Autodesk Fusion 360 part; units mm, degrees
(part 3 of 3)
  point P128 (211, 51)
  point P129 (218.0002, 50.9466)
  point P130 (228.5461, 44.9647)
  point P131 (221.5464, 44.9113)
  point P132 (225, 51)
  point P133 (225, 51)
  point P134 (225, 51)
  point P135 (134.0002, 62.9466)
  point P136 (144.5461, 56.9647)
  point P137 (137.5464, 56.9113)
  point P138 (141, 63)
  point P139 (141, 63)
  point P140 (141, 63)
  point P141 (148.0002, 62.9466)
  point P142 (158.5461, 56.9647)
  point P143 (151.5464, 56.9113)
  point P144 (155, 63)
  point P145 (155, 63)
  point P146 (155, 63)
  point P147 (162.0002, 62.9466)
  point P148 (172.5461, 56.9647)
  point P149 (165.5464, 56.9113)
  point P150 (169, 63)
  point P151 (169, 63)
  point P152 (169, 63)
  point P153 (190.0002, 62.9466)
  point P154 (200.5461, 56.9647)
  point P155 (193.5464, 56.9113)
  point P156 (197, 63)
  point P157 (197, 63)
  point P158 (197, 63)
  point P159 (204.0002, 62.9466)
  point P160 (214.5461, 56.9647)
  point P161 (207.5464, 56.9113)
  point P162 (211, 63)
  point P163 (211, 63)
  point P164 (211, 63)
  point P165 (218.0002, 62.9466)
  point P166 (228.5461, 56.9647)
  point P167 (221.5464, 56.9113)
  point P168 (225, 63)
  point P169 (225, 63)
  point P170 (225, 63)
  point P171 (134.0002, 74.9466)
  point P172 (144.5461, 68.9647)
  point P173 (137.5464, 68.9113)
  point P174 (141, 75)
  point P175 (141, 75)
  point P176 (141, 75)
  point P177 (148.0002, 74.9466)
  point P178 (158.5461, 68.9647)
  point P179 (151.5464, 68.9113)
  point P180 (155, 75)
  point P181 (155, 75)
  point P182 (155, 75)
  point P183 (162.0002, 74.9466)
  point P184 (172.5461, 68.9647)
  point P185 (165.5464, 68.9113)
  point P186 (169, 75)
  point P187 (169, 75)
  point P188 (169, 75)
  point P189 (176.0002, 74.9466)
  point P190 (186.5461, 68.9647)
  point P191 (179.5464, 68.9113)
  point P192 (183, 75)
  point P193 (183, 75)
  point P194 (183, 75)
  point P195 (190.0002, 74.9466)
  point P196 (200.5461, 68.9647)
  point P197 (193.5464, 68.9113)
  point P198 (197, 75)
  point P199 (197, 75)
  point P200 (197, 75)
  point P201 (204.0002, 74.9466)
  point P202 (214.5461, 68.9647)
  point P203 (207.5464, 68.9113)
  point P204 (211, 75)
  point P205 (211, 75)
  point P206 (211, 75)
  point P207 (218.0002, 74.9466)
  point P208 (228.5461, 68.9647)
  point P209 (221.5464, 68.9113)
  point P210 (225, 75)
  point P211 (225, 75)
  point P212 (225, 75)
  point P213 (134.0002, 86.9466)
  point P214 (144.5461, 80.9647)
  point P215 (137.5464, 80.9113)
  point P216 (141, 87)
  point P217 (141, 87)
  point P218 (141, 87)
  point P219 (148.0002, 86.9466)
  point P220 (158.5461, 80.9647)
  point P221 (151.5464, 80.9113)
  point P222 (155, 87)
  point P223 (155, 87)
  point P224 (155, 87)
  point P225 (162.0002, 86.9466)
  point P226 (172.5461, 80.9647)
  point P227 (165.5464, 80.9113)
  point P228 (169, 87)
  point P229 (169, 87)
  point P230 (169, 87)
  point P231 (176.0002, 86.9466)
  point P232 (186.5461, 80.9647)
  point P233 (179.5464, 80.9113)
  point P234 (183, 87)
  point P235 (183, 87)
  point P236 (183, 87)
  point P237 (190.0002, 86.9466)
  point P238 (200.5461, 80.9647)
  point P239 (193.5464, 80.9113)
  point P240 (197, 87)
  point P241 (197, 87)
  point P242 (197, 87)
  point P243 (204.0002, 86.9466)
  point P244 (214.5461, 80.9647)
  point P245 (207.5464, 80.9113)
  point P246 (211, 87)
  point P247 (211, 87)
  point P248 (211, 87)
  point P249 (218.0002, 86.9466)
  point P250 (228.5461, 80.9647)
  point P251 (221.5464, 80.9113)
  point P252 (225, 87)
  point P253 (225, 87)
  point P254 (225, 87)
  point P255 (134.0002, 98.9466)
  point P256 (144.5461, 92.9647)
  point P257 (137.5464, 92.9113)
  point P258 (141, 99)
  point P259 (141, 99)
  point P260 (141, 99)
  point P261 (148.0002, 98.9466)
  point P262 (158.5461, 92.9647)
  point P263 (151.5464, 92.9113)
  point P264 (155, 99)
  point P265 (155, 99)
  point P266 (155, 99)
  point P267 (162.0002, 98.9466)
  point P268 (172.5461, 92.9647)
  point P269 (165.5464, 92.9113)
  point P270 (169, 99)
  point P271 (169, 99)
  point P272 (169, 99)
  point P273 (176.0002, 98.9466)
  point P274 (186.5461, 92.9647)
  point P275 (179.5464, 92.9113)
  point P276 (183, 99)
  point P277 (183, 99)
  point P278 (183, 99)
  point P279 (190.0002, 98.9466)
  point P280 (200.5461, 92.9647)
  point P281 (193.5464, 92.9113)
  point P282 (197, 99)
  point P283 (197, 99)
  point P284 (197, 99)
  point P285 (204.0002, 98.9466)
  point P286 (214.5461, 92.9647)
  point P287 (207.5464, 92.9113)
  point P288 (211, 99)
  point P289 (211, 99)
  point P290 (211, 99)
  point P291 (218.0002, 98.9466)
  point P292 (228.5461, 92.9647)
  point P293 (221.5464, 92.9113)
  point P294 (225, 99)
  point P295 (225, 99)
  point P296 (225, 99)
  dimension "d52" = 75
  dimension "d55" = 3
  dimension "d56" = 3
  dimension "d57" = 3
  dimension "d58" = 3
  dimension "d59" = 1
  dimension "d60" = 1
  dimension "d61" = 1
  dimension "d62" = 1
  dimension "d63" = 1
  dimension "d64" = 60
  dimension "d65" = 60
  dimension "d68" = 42
  dimension "d69" = 36
  constraint coincident L10.end L11.start
  constraint coincident L13.end L15.start
  constraint coincident P5 A0.centre
  constraint parallel L54 L71
  constraint parallel L63 L65
  constraint coincident A0 L77.end
  constraint perpendicular L58 L77
  measures "d52" diameter of A0
  measures "d55" distance of P5 L58
  measures "d56" distance of P6 L64
  measures "d57" distance of P7 L70
  measures "d58" distance of P8 L76
  measures "d59" distance of L58 L64
  measures "d60" distance of L54 L71
  measures "d61" distance of L63 L65
  measures "d62" distance of L53 L70
  measures "d63" distance of L69 L72
  measures "d64" distance of P5 L52
  measures "d65" distance of L23 P5
extrude "Extrude5" add sketch "Sketch4" along normal blind 6 separate body contours A0 L127 L130 L147 L151 L154 L155 L159 L162 L168 L169 L171 L175 L178 L179 L183 L186 L192 L193 L271 L274 L278 L287 L291 L292 L293 L294 L296 L304 L305 L309 L349 L350 L356 L364 L365 L367 L368 L370 L377 L378 L381 L382 L438 L447 L448 L449 L451 L453 L456 L457 L541 L542 L548 L557 L561 L563 L567 L577 L588 L604 L605 L609 L615 L619 L624 L625 L704 L705 L707 L711 L715 L717 L721 L722 L732 L748 L749 L753 L759 L763 L768 L872 L873 L875 L883 L885 L889 L890 L913 L914 L922 L923 L928 L929 L932 L933 L1012 L1014 L1015 L1016 L1020 L1022 L1024 L1025 L1073 L1080 L1088 L1090 L1092 L1100 L1101 L1106 L1107 L1110 L1111 L1117 L1119 L1126 L1127 L1130 L1131 L1132 L1135 L1141 L1143 L1144 L1145 L1146 L1150 L1151 L1152 L1154 L1155 L1156 L1160 L1164 L1172 L1182 makes body 5
extrude "Extrude6" add sketch "Sketch4" along normal blind 6 contours L0 L1 L2 L3 L4 L5 L6 L7 L8 L9 L10 L11 L12 L13 L14 L15 L16 L17 L18 L19 L20 L21 L22 L23 L24 L25 L26 L27 L28 L29 L30 L31 L32 L33 L34 L35 L36 L37 L38 L39 L40 L41 L42 L43 L44 L45 L46 L47 L48 L49 L50 L51 | A0 L1091 L1094 L1102 L1106 L1111 | A0 L276 L277 L278 L284 L292 | A0 L1074 L1075 L1080 L1088 L1089 | A0 L274 L282 L286 L287 | A0 L914 L917 L924 L928 | A0 L440 L448 L453 L458 | A0 L915 L923 L927 L932 | A0 L441 L443 L451 L457 | A0 L753 L755 L759 L769 | A0 L588 L589 L590 L596 L605 | A0 L732 L733 L734 L740 L749 | A0 L609 L611 L625 | L79 L82 L90 L94 L95 L99 | L81 L83 L87 L91 L96 L97 | L246 L248 L256 L257 L261 L266 | L247 L250 L258 L262 L263 L267 | L249 L251 L255 L259 L264 L265 | L252 L253 L254 L260 L268 L269 | L270 L272 L280 L281 L285 L290 | L273 L275 L279 L283 L288 L289 | L414 L416 L424 L425 L429 L434 | L415 L418 L426 L430 L431 L435 | L417 L419 L423 L427 L432 L433 | L420 L421 L422 L428 L436 L437 | L582 L584 L592 L593 L597 L602 | L583 L586 L594 L598 L599 L603 | L585 L587 L591 L595 L600 L601 | L726 L728 L736 L737 L741 L746 | L727 L730 L738 L742 L743 L747 | L729 L731 L735 L739 L744 L745 | L894 L895 L902 L903 L907 L910 | L896 L898 L901 L905 L908 L909 | L1067 L1069 L1076 L1077 L1081 L1086 | L1068 L1071 L1078 L1082 L1083 L1087 | L1093 L1095 L1099 L1103 L1108 L1109 bodies 5
extrude "Extrude7" add sketch "Sketch4" along normal blind 6 contours A0 L175 L186 L190 L191 L195 | A0 L177 L179 L187 L192 | A0 L162 L166 L167 L171 | A0 L153 L155 L163 L168 | A0 L130 L138 L142 L143 L147 | L78 L80 L88 L89 L93 L98 | L84 L85 L86 L92 L100 L101 | L102 L104 L112 L113 L117 L122 | L103 L106 L114 L118 L119 L123 | L105 L107 L111 L115 L120 L121 | L108 L109 L110 L116 L124 L125 | L126 L128 L136 L137 L141 L146 | L129 L131 L135 L139 L144 L145 | L132 L133 L134 L140 L148 L149 | L150 L152 L160 L161 L165 L170 | L156 L157 L158 L164 L172 L173 | L174 L176 L184 L185 L189 L194 | L180 L181 L182 L188 L196 L197 | L198 L200 L208 L209 L213 L218 | L199 L202 L210 L214 L215 L219 | L201 L203 L207 L211 L216 L217 | L204 L205 L206 L212 L220 L221 bodies 5
extrude "Extrude8" add sketch "Sketch4" along normal blind 6 contours A0 L711 L715 L720 | A0 L702 L712 L713 L717 L722 | A0 L870 L880 L881 L885 L890 | A0 L561 L567 L571 L576 | A0 L879 L883 L888 L889 | A0 L540 L548 L556 L557 | A0 L1014 L1016 L1030 L1031 | A0 L367 L382 L383 L387 | A0 L1009 L1012 L1025 L1029 | A0 L366 L368 L376 L377 L386 | A0 L1162 L1164 L1172 L1173 L1177 | A0 L1139 L1142 L1150 L1155 L1159 | A0 L1143 L1147 L1156 L1157 | A0 L1115 L1118 L1126 L1135 | A0 L1119 L1123 L1132 L1133 | L222 L224 L232 L233 L237 L242 | L223 L226 L234 L238 L239 L243 | L225 L227 L231 L235 L240 L241 | L228 L229 L230 L236 L244 L245 | L372 L373 L374 L380 L388 L389 | L390 L392 L400 L401 L405 L410 | L391 L394 L402 L406 L407 L411 | L393 L395 L399 L403 L408 L409 | L396 L397 L398 L404 L412 L413 | L558 L560 L568 L569 L573 L578 | L559 L562 L570 L574 L575 L579 | L564 L565 L566 L572 L580 L581 | L703 L706 L714 L718 L719 L723 | L708 L709 L710 L716 L724 L725 | L871 L874 L882 L886 L887 L891 | L876 L877 L878 L884 L892 L893 | L1032 L1034 L1042 L1043 L1047 L1052 | L1033 L1036 L1044 L1048 L1049 L1053 | L1035 L1037 L1041 L1045 L1050 L1051 | L1038 L1039 L1040 L1046 L1054 L1055 | L1163 L1166 L1174 L1178 L1179 L1183 | L1165 L1167 L1171 L1175 L1180 L1181 | L1168 L1169 L1170 L1176 L1184 L1185 | L1186 L1188 L1196 L1197 L1201 L1206 | L1187 L1190 L1198 L1202 L1203 L1207 | L1189 L1191 L1195 L1199 L1204 L1205 | L1192 L1193 L1194 L1200 L1208 L1209 bodies 5
copy_body "Body->Comp1" bodies 5 removing the originals makes body 6 in component "Component"
sketch "Sketch5" plane through (0, 0, 6) normal (0, 0, 1) x (-1, 0, 0)
  line L0 (-105.9375, -126) -> (-120, -126)
  line L1 (-120, -126) -> (-120, -140.0625)
  line L2 (-120, -140.0625) -> (-117, -140.0625)
  line L3 (-117, -140.0625) -> (-117, -158.4375)
  line L4 (-117, -158.4375) -> (-120, -158.4375)
  line L5 (-120, -158.4375) -> (-120, -176.8125)
  line L6 (-120, -176.8125) -> (-117, -176.8125)
  line L7 (-117, -176.8125) -> (-117, -195.1875)
  line L8 (-117, -195.1875) -> (-120, -195.1875)
  line L9 (-120, -195.1875) -> (-120, -213.5625)
  line L10 (-120, -213.5625) -> (-117, -213.5625)
  line L11 (-117, -213.5625) -> (-117, -231.9375)
  line L12 (-117, -231.9375) -> (-120, -231.9375)
  line L13 (-120, -231.9375) -> (-120, -246)
  line L14 (-120, -246) -> (-105.9375, -246)
  line L15 (-105.9375, -246) -> (-105.9375, -243)
  line L16 (-105.9375, -243) -> (-87.5625, -243)
  line L17 (-87.5625, -243) -> (-87.5625, -246)
  line L18 (-87.5625, -246) -> (-69.1875, -246)
  line L19 (-69.1875, -246) -> (-69.1875, -243)
  line L20 (-69.1875, -243) -> (-50.8125, -243)
  line L21 (-50.8125, -243) -> (-50.8125, -246)
  line L22 (-50.8125, -246) -> (-32.4375, -246)
  line L23 (-32.4375, -246) -> (-32.4375, -243)
  line L24 (-32.4375, -243) -> (-14.0625, -243)
  line L25 (-14.0625, -243) -> (-14.0625, -246)
  line L26 (-14.0625, -246) -> (0, -246)
  line L27 (0, -246) -> (0, -231.9375)
  line L28 (0, -231.9375) -> (-3, -231.9375)
  line L29 (-3, -231.9375) -> (-3, -213.5625)
  line L30 (-3, -213.5625) -> (0, -213.5625)
  line L31 (0, -213.5625) -> (0, -195.1875)
  line L32 (0, -195.1875) -> (-3, -195.1875)
  line L33 (-3, -195.1875) -> (-3, -176.8125)
  line L34 (-3, -176.8125) -> (0, -176.8125)
  line L35 (0, -176.8125) -> (0, -158.4375)
  line L36 (0, -158.4375) -> (-3, -158.4375)
  line L37 (-3, -158.4375) -> (-3, -140.0625)
  line L38 (-3, -140.0625) -> (0, -140.0625)
  line L39 (0, -140.0625) -> (0, -126)
  line L40 (0, -126) -> (-14.0625, -126)
  line L41 (-14.0625, -126) -> (-14.0625, -129)
  line L42 (-14.0625, -129) -> (-32.4375, -129)
  line L43 (-32.4375, -129) -> (-32.4375, -126)
  line L44 (-32.4375, -126) -> (-50.8125, -126)
  line L45 (-50.8125, -126) -> (-50.8125, -129)
  line L46 (-50.8125, -129) -> (-69.1875, -129)
  line L47 (-69.1875, -129) -> (-69.1875, -126)
  line L48 (-69.1875, -126) -> (-87.5625, -126)
  line L49 (-87.5625, -126) -> (-87.5625, -129)
  line L50 (-87.5625, -129) -> (-105.9375, -129)
  line L51 (-105.9375, -129) -> (-105.9375, -126)
  line L52 (-50.8125, -126) -> (-69.1875, -126) construction
  circle A0 centre (-60, -156) radius 10
  line L53 (-60, -126) -> (-60, -156) construction
  dimension "d78" = 20
  dimension "d83" = 30
  constraint coincident L44.end L45.start
  constraint coincident L47.end L48.start
  constraint midpoint L52 L53.start
  constraint perpendicular L52 L53
  constraint coincident A0.centre L53.end
  measures "d78" diameter of A0
  measures "d83" distance of L53.start A0.centre
extrude "Extrude9" cut sketch "Sketch5" against normal blind 6 contours A0 bodies 4
component "Component" placed x (1, 0, 0) y (0, 1, 0) z (0, 0, 1) at (0, 0, 0)
component "Component" placed x (1, 0, 0) y (0, 1, 0) z (0, 0, 1) at (0, 123, 0)
equation "d1 = button_diameter"
equation "d4 = button_diameter"
equation "d7 = button_diameter"
equation "d10 = button_diameter"
equation "d13 = thickness"
equation "d46 = thickness"
equation "d48 = thickness"
equation "d50 = thickness"
equation "d52 = speaker_diameter"
equation "d70 = thickness"
equation "d72 = thickness"
equation "d74 = thickness"
equation "d76 = thickness"
equation "d78 = wirehole_diameter"
equation "thickness = 6 mm"
equation "wirehole_diameter = 20 mm"
equation "d81 = -thickness"
equation "button_diameter = 30 mm"
equation "speaker_diameter = 75 mm"
